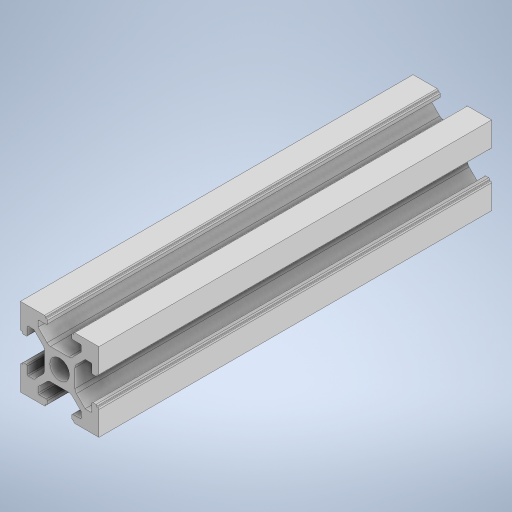
# Autodesk Inventor part: T slot beam 20mm Dist_40mm
Saved by Autodesk Inventor 2023.5 (Build 275446000, 446)
## iProperties
Created: 2024-07-24
Part Number: T slot beam 20mm Dist_40mm
Material: Generic
Document SubType Name: Modeling
Designer: Big Sean T
Density: 1 g/cm^3
Appearance: Default
Author: Big Sean T
Autodesk Inventor part; units mm, degrees
ref_plane "YZ Plane" through (0, 0, 0) normal (1, 0, 0) x (0, 1, 0)
ref_plane "XZ Plane" through (0, 0, 0) normal (0, 1, 0) x (-1, 0, 0)
ref_plane "XY Plane" through (0, 0, 0) normal (0, 0, 1) x (1, 0, 0)
sketch "Sketch1" plane through (0, 0, 0) normal (0, 0, 1) x (1, 0, 0)
  line L0 (0, 0) -> (6.146, 0)
  line L1 (6.4, 0.254) -> (6.4, 0.5)
  line L2 (6.4, 0.5) -> (6.646, 0.5)
  line L3 (6.9, 0.754) -> (6.9, 1.546)
  line L4 (0, 0) -> (0, 6.146)
  line L5 (0.254, 6.4) -> (0.5, 6.4)
  line L6 (0.5, 6.4) -> (0.5, 6.646)
  line L7 (0.754, 6.9) -> (1.5449, 6.9)
  line L8 (1.7989, 6.646) -> (1.7989, 4.8147)
  line L9 (6.646, 1.8) -> (4.754, 1.8)
  line L10 (20, 0) -> (20, 6.146)
  line L11 (19.746, 6.4) -> (19.5, 6.4)
  line L12 (19.5, 6.4) -> (19.5, 6.646)
  line L13 (19.246, 6.9) -> (18.4551, 6.9)
  line L14 (18.2011, 6.646) -> (18.2011, 4.8147)
  line L15 (20, 0) -> (13.854, 0)
  line L16 (13.6, 0.254) -> (13.6, 0.5)
  circle A0 centre (10, 10) radius 2.5
  line L17 (20, 20) -> (13.854, 20)
  line L18 (20, 20) -> (20, 13.854)
  line L19 (19.746, 13.6) -> (19.5, 13.6)
  line L20 (19.5, 13.6) -> (19.5, 13.354)
  line L21 (19.246, 13.1) -> (18.454, 13.1)
  line L22 (13.6, 19.746) -> (13.6, 19.5)
  line L23 (13.6, 19.5) -> (13.354, 19.5)
  line L24 (13.1, 19.246) -> (13.1, 18.454)
  line L25 (13.354, 18.2) -> (15.246, 18.2)
  line L26 (0, 20) -> (6.146, 20)
  line L27 (6.4, 19.746) -> (6.4, 19.5)
  line L28 (6.4, 19.5) -> (6.646, 19.5)
  line L29 (6.9, 19.246) -> (6.9, 18.454)
  line L30 (6.646, 18.2) -> (4.754, 18.2)
  line L31 (0, 20) -> (0, 13.854)
  line L32 (0.254, 13.6) -> (0.5, 13.6)
  line L33 (0.5, 13.6) -> (0.5, 13.354)
  line L34 (0.754, 13.1) -> (1.546, 13.1)
  line L35 (1.8, 13.354) -> (1.8, 15.246)
  line L36 (3.4393, 15.5) -> (2.054, 15.5)
  line L37 (4.5, 16.5607) -> (4.5, 17.946)
  line L38 (16.5, 4.5607) -> (17.9471, 4.5607)
  line L39 (13.6, 0.5) -> (13.354, 0.5)
  line L40 (13.1, 0.754) -> (13.1, 1.546)
  line L41 (13.354, 1.8) -> (15.246, 1.8)
  line L42 (15.5, 2.054) -> (15.5, 3.4393)
  line L43 (15.5, 16.5607) -> (15.5, 17.946)
  line L44 (16.5, 15.4393) -> (17.946, 15.4393)
  line L45 (4.5, 3.4393) -> (4.5, 2.054)
  line L46 (3.5, 4.5607) -> (2.0529, 4.5607)
  line L47 (6.1, 7.6867) -> (6.1, 12.3133)
  line L48 (3.5, 4.5607) -> (5.728, 6.7887)
  line L49 (3.4393, 15.5) -> (5.728, 13.2113)
  line L50 (7.6867, 13.9) -> (12.3133, 13.9)
  line L51 (6.7887, 14.272) -> (4.5, 16.5607)
  line L52 (13.2113, 14.272) -> (15.5, 16.5607)
  line L53 (13.9, 12.3133) -> (13.9, 7.6867)
  line L54 (14.272, 6.7887) -> (16.5, 4.5607)
  line L55 (14.272, 13.2113) -> (16.5, 15.4393)
  line L56 (7.6867, 6.1) -> (12.3133, 6.1)
  line L57 (6.7887, 5.728) -> (4.5, 3.4393)
  line L58 (13.2113, 5.728) -> (15.5, 3.4393)
  arc A1 (6.9, 19.246) -> (6.646, 19.5) centre (6.646, 19.246) ccw
  arc A2 (6.4, 19.746) -> (6.146, 20) centre (6.146, 19.746) ccw
  arc A3 (6.646, 18.2) -> (6.9, 18.454) centre (6.646, 18.454) ccw
  arc A4 (4.754, 18.2) -> (4.5, 17.946) centre (4.754, 17.946) ccw
  arc A5 (13.1, 18.454) -> (13.354, 18.2) centre (13.354, 18.454) ccw
  arc A6 (13.354, 19.5) -> (13.1, 19.246) centre (13.354, 19.246) ccw
  arc A7 (13.854, 20) -> (13.6, 19.746) centre (13.854, 19.746) ccw
  arc A8 (15.5, 17.946) -> (15.246, 18.2) centre (15.246, 17.946) ccw
  arc A9 (2.054, 15.5) -> (1.8, 15.246) centre (2.054, 15.246) ccw
  arc A10 (0.5, 13.354) -> (0.754, 13.1) centre (0.754, 13.354) ccw
  arc A11 (0, 13.854) -> (0.254, 13.6) centre (0.254, 13.854) ccw
  arc A12 (1.546, 13.1) -> (1.8, 13.354) centre (1.546, 13.354) ccw
  arc A13 (0.254, 6.4) -> (0, 6.146) centre (0.254, 6.146) ccw
  arc A14 (0.754, 6.9) -> (0.5, 6.646) centre (0.754, 6.646) ccw
  arc A15 (1.7989, 6.646) -> (1.5449, 6.9) centre (1.5449, 6.646) ccw
  arc A16 (1.7989, 4.8147) -> (2.0529, 4.5607) centre (2.0529, 4.8147) ccw
  arc A17 (19.746, 13.6) -> (20, 13.854) centre (19.746, 13.854) ccw
  arc A18 (19.246, 13.1) -> (19.5, 13.354) centre (19.246, 13.354) ccw
  arc A19 (18.2, 13.354) -> (18.454, 13.1) centre (18.454, 13.354) ccw
  line L59 (18.2, 13.354) -> (18.2, 15.1853)
  arc A20 (18.2, 15.1853) -> (17.946, 15.4393) centre (17.946, 15.1853) ccw
  arc A21 (20, 6.146) -> (19.746, 6.4) centre (19.746, 6.146) ccw
  arc A22 (19.5, 6.646) -> (19.246, 6.9) centre (19.246, 6.646) ccw
  arc A23 (18.4551, 6.9) -> (18.2011, 6.646) centre (18.4551, 6.646) ccw
  arc A24 (17.9471, 4.5607) -> (18.2011, 4.8147) centre (17.9471, 4.8147) ccw
  arc A25 (13.6, 0.254) -> (13.854, 0) centre (13.854, 0.254) ccw
  arc A26 (13.1, 0.754) -> (13.354, 0.5) centre (13.354, 0.754) ccw
  arc A27 (13.354, 1.8) -> (13.1, 1.546) centre (13.354, 1.546) ccw
  arc A28 (15.246, 1.8) -> (15.5, 2.054) centre (15.246, 2.054) ccw
  arc A29 (6.146, 0) -> (6.4, 0.254) centre (6.146, 0.254) ccw
  arc A30 (6.646, 0.5) -> (6.9, 0.754) centre (6.646, 0.754) ccw
  arc A31 (6.9, 1.546) -> (6.646, 1.8) centre (6.646, 1.546) ccw
  arc A32 (4.5, 2.054) -> (4.754, 1.8) centre (4.754, 2.054) ccw
  arc A33 (6.7887, 14.272) -> (7.6867, 13.9) centre (7.6867, 15.17) ccw
  arc A34 (12.3133, 13.9) -> (13.2113, 14.272) centre (12.3133, 15.17) ccw
  arc A35 (6.1, 12.3133) -> (5.728, 13.2113) centre (4.83, 12.3133) ccw
  arc A36 (5.728, 6.7887) -> (6.1, 7.6867) centre (4.83, 7.6867) ccw
  arc A37 (7.6867, 6.1) -> (6.7887, 5.728) centre (7.6867, 4.83) ccw
  arc A38 (13.2113, 5.728) -> (12.3133, 6.1) centre (12.3133, 4.83) ccw
  arc A39 (13.9, 7.6867) -> (14.272, 6.7887) centre (15.17, 7.6867) ccw
  arc A40 (14.272, 13.2113) -> (13.9, 12.3133) centre (15.17, 12.3133) ccw
  point P0 (20, 6.4)
  point P1 (19.5, 6.9)
  point P2 (18.2011, 6.9)
  dimension "d59" = 1.27
  constraints: 120 end point, 80 point on circle, 79 tangent, 41 centre point, 37 equal radius, 32 perpendicular, 12 point on line, 6 horizontal, 2 vertical, 1 collinear, 1 parallel
  measures "d59" radius of A33
extrude "Extrusion1" add sketch "Sketch1" along normal blind 100
body "Solid1"
